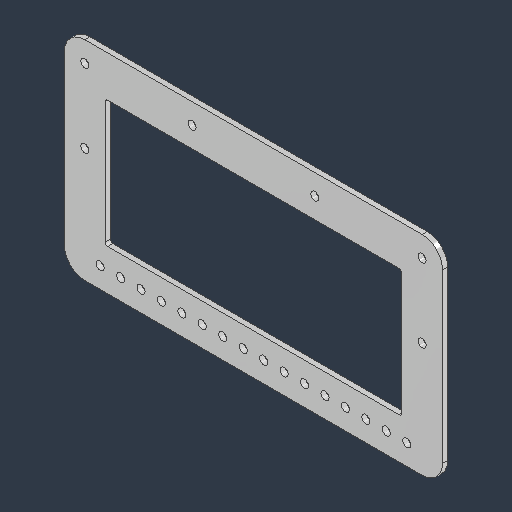
# Autodesk Inventor part: PLATE,MOUNT,BATTERY,TOP
Saved by Autodesk Inventor 2024.3 (Build 283343000, 343)
## iProperties
ILogicPurgeVersion: 0.0.0.0
OnSaveVersion: 3.4.3.0
OnSaveAssembly: COREAutomationManager
Created: 2025-01-28
Part Number: PLATE,MOUNT,BATTERY,TOP
Material: Aluminum 3003-O
Document SubType Name: Sheet Metal
Designer: Jthib
Density: 2.73809 g/cm^3
Sheet Metal Rule: Default
Appearance: Aluminum - Polished
Mass: 133.434 g
Surface Area: 357.239 cm^2
Volume: 48.7324 cm^3
Mfg Approved By: John.Thibert
ModelCat: Uncategorized
MaterialName: Aluminum 3003-O
CN_MASS: 0.13
Author: Jthib
Autodesk Inventor part; units mm, degrees
ref_plane "YZ Plane" through (0, 0, 0) normal (1, 0, 0) x (0, 1, 0)
ref_plane "XZ Plane" through (0, 0, 0) normal (0, 1, 0) x (-1, 0, 0)
ref_plane "XY Plane" through (0, 0, 0) normal (0, 0, 1) x (1, 0, 0)
sketch "Sketch1" plane through (0, 0, 0) normal (0, 0, 1) x (1, 0, 0)
  line L0 (-92.075, -39.37) -> (92.075, -39.37)
  line L1 (92.075, -39.37) -> (92.075, 39.37)
  line L2 (92.075, 39.37) -> (-92.075, 39.37)
  line L3 (-92.075, 39.37) -> (-92.075, -39.37)
  line L4 (-92.075, -39.37) -> (92.075, 39.37) construction
  line L5 (92.075, -39.37) -> (-92.075, 39.37) construction
  line L6 (-117.475, 64.77) -> (117.475, 64.77)
  line L7 (117.475, 64.77) -> (117.475, -64.77)
  line L8 (117.475, -64.77) -> (-117.475, -64.77)
  line L9 (-117.475, -64.77) -> (-117.475, 64.77)
  point P0 (0, 0)
  dimension "d0" = 184.15
  dimension "d1" = 78.74
  dimension "d2" = 25.4
  measures "d0" distance of L1.end L2.end
  measures "d1" distance of L2.end L0.start
  measures "d2" distance between parallel lines of L2 L6
extrude "Plate1" add sketch "Sketch1" along normal mid plane 3.175
sketch "Sketch2" plane through (0, 0, 1.5875) normal (0, 0, 1) x (1, 0, 0)
  line L0 (-92.075, -39.37) -> (-92.075, 39.37) construction
  line L1 (-92.075, 39.37) -> (92.075, 39.37) construction
  line L2 (92.075, 39.37) -> (92.075, -39.37) construction
  line L3 (92.075, -39.37) -> (-92.075, -39.37) construction
  line L4 (104.775, 52.07) -> (-104.775, 52.07) construction
  line L5 (-104.775, 52.07) -> (-104.775, -52.07) construction
  line L6 (-104.775, -52.07) -> (104.775, -52.07) construction
  line L7 (104.775, -52.07) -> (104.775, 52.07) construction
  line L8 (0, 90.678) -> (0, -90.678) construction
  point P0 (0, 0)
  point P1 (-95.25, -52.07)
  point P2 (-82.55, -52.07)
  point P3 (-69.85, -52.07)
  point P4 (-57.15, -52.07)
  point P5 (-44.45, -52.07)
  point P6 (-31.75, -52.07)
  point P7 (-19.05, -52.07)
  point P8 (-6.35, -52.07)
  point P9 (6.35, -52.07)
  point P10 (19.05, -52.07)
  point P11 (31.75, -52.07)
  point P12 (44.45, -52.07)
  point P13 (57.15, -52.07)
  point P14 (69.85, -52.07)
  point P15 (82.55, -52.07)
  point P16 (95.25, -52.07)
  point P17 (-38.1, 52.07)
  point P18 (38.1, 52.07)
  point P19 (-104.775, 6.35)
  point P20 (104.775, 6.35)
  dimension "d4" = 12.7
  dimension "d16" = 12.7
  dimension "d21" = 9.525
  dimension "d22" = 9.525
  dimension "d23" = 66.675
  dimension "d24" = 66.675
  dimension "d25" = 76.2
  dimension "d26" = 45.72
  dimension "d28" = 45.72
  constraints: 8 end point, 5 point on line, 2 coincident, 1 horizontal, 18 other
  measures "d4" distance between parallel lines of L4 L1
  measures "d16" distance of point (-95.25, -52.07) point (-82.55, -52.07)
  measures "d21" distance from line of L5 point (-95.25, -52.07)
  measures "d22" distance from line of L7 point (95.25, -52.07)
  measures "d23" distance of L4.end point (-38.1, 52.07)
  measures "d24" distance of point (104.775, 52.07) point (38.1, 52.07)
  measures "d25" distance of point (38.1, 52.07) point (-38.1, 52.07)
  measures "d26" distance of point (-104.775, 52.07) point (-104.775, 6.35)
  measures "d28" distance from line of L4 point (104.775, 6.35)
hole "Hole1" at (-104.775, 52.07, 1.5875) at (104.775, 52.07, 1.5875) at (-95.25, -52.07, 1.5875) at (-82.55, -52.07, 1.5875) at (-69.85, -52.07, 1.5875) at (-57.15, -52.07, 1.5875) at (-44.45, -52.07, 1.5875) at (-31.75, -52.07, 1.5875) at (-19.05, -52.07, 1.5875) at (-6.35, -52.07, 1.5875) at (6.35, -52.07, 1.5875) at (19.05, -52.07, 1.5875) at (31.75, -52.07, 1.5875) at (44.45, -52.07, 1.5875) at (57.15, -52.07, 1.5875) at (69.85, -52.07, 1.5875) at (82.55, -52.07, 1.5875) at (95.25, -52.07, 1.5875) at (-38.1, 52.07, 1.5875) at (38.1, 52.07, 1.5875) at (-104.775, 6.35, 1.5875) at (104.775, 6.35, 1.5875) direction (0, 0, -1) diameter 5.1054 end through all clearance for "Flat Head Machine Screw (82)" size "#10" standard "Ansi Unified Screw Threads"
fillet "Corner Round1" radius 1.5875 4 edges at (-92.075, -39.37, 0) (-92.075, 39.37, 0) (92.075, 39.37, 0) (92.075, -39.37, 0)
fillet "Corner Round2" radius 12.7 4 edges at (-117.475, 64.77, 0) (117.475, 64.77, 0) (117.475, -64.77, 0) (-117.475, -64.77, 0)
equation "\"d21\" = d22"
equation "\"d23\" = d24"
equation "\"d28\" = d26"
equation "\"d34\" = Thickness"
equation "\"d3\" = Thickness"
equation "\"BendRadius\" = Thickness"
equation "\"BendReliefWidth\" = Thickness"
equation "\"BendReliefDepth\" = 0.5 * Thickness"
equation "\"CornerReliefSize\" = 4 * Thickness"
equation "\"MinimumRemnant\" = 2 * Thickness"
equation "\"TransitionRadius\" = BendRadius"
equation "\"JacobiRadiusSize\" = BendRadius"
equation "\"GapSize\" = Thickness"
equation "\"Thickness\" = 3.175"
body "Solid1"
